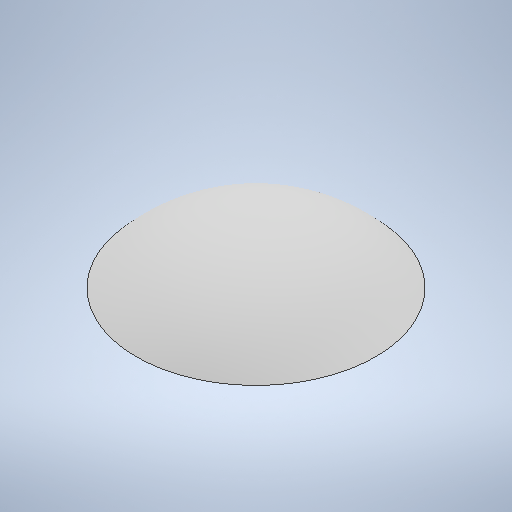
# Autodesk Inventor part: case_chaleco
Saved by Autodesk Inventor 2025.2 (Build 292293000, 293)
## iProperties
Created: 2026-03-17
Part Number: case_chaleco
Material: Genérico
Document SubType Name: Modeling
Designer: Periscopio
Density: 1 g/cm^3
Appearance: Valor por defecto
Author: Periscopio
Autodesk Inventor part; units mm, degrees
ref_plane "YZ Plane" through (0, 0, 0) normal (1, 0, 0) x (0, 1, 0)
ref_plane "XZ Plane" through (0, 0, 0) normal (0, 1, 0) x (-1, 0, 0)
ref_plane "XY Plane" through (0, 0, 0) normal (0, 0, 1) x (1, 0, 0)
sketch "Boceto1" plane through (0, 0, 0) normal (1, 0, 0) x (0, 1, 0)
  line L0 (0, 0) -> (0, -65)
  line L1 (0, 0) -> (30, 0)
  arc A0 (0, -65) -> (30, 0) centre (-54.1898, -0.5663) ccw
  dimension "d0" = 65
  dimension "d1" = 30
  constraints: 4 end point, 2 point on circle, 1 centre point, 1 horizontal, 1 vertical
  measures "d0" distance of L0.start L0.end
  measures "d1" distance of L0.start L1.end
revolve "Revolución1" add sketch "Boceto1" angle 360 about axis through (0, 0, 0) along (0, 1, 0)
